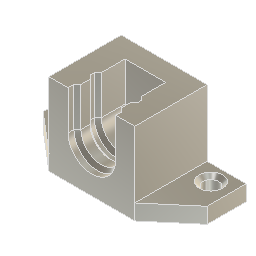
Крепление пневматического инструмента (Autodesk Fusion 360 design; units mm, degrees)
Autodesk Fusion 360 part; units mm, degrees
sketch "Sketch1" plane through (0, 0, 0) normal (0, 0, 1) x (1, 0, 0)
  line L0 (-5.9, 3.5) -> (-11, 3.5)
  line L1 (-11, 3.5) -> (-11, 22)
  line L2 (-11, 22) -> (0, 22)
  line L3 (5.9, 3.5) -> (11, 3.5)
  line L4 (11, 22) -> (0, 22)
  line L5 (11, 3.5) -> (11, 22)
  line L6 (-5.9, 3.5) -> (5.9, 3.5)
  line L7 (-6.1, 4.9828) -> (-6.1, 3.5)
  line L8 (-5.2, 5.8828) -> (-6.1, 4.9828)
  line L9 (-5.2, 8.2172) -> (-5.2, 5.8828)
  line L10 (-6.1, 9.1172) -> (-5.2, 8.2172)
  line L11 (-6.1, 9.1172) -> (-6.1, 10.1828)
  line L12 (-5.2, 11.0828) -> (-6.1, 10.1828)
  line L13 (-5.2, 16) -> (-5.2, 11.0828)
  line L14 (-5.2, 16) -> (-5.2, 17.2)
  line L15 (-5.2, 17.2) -> (0, 17.2)
  line L16 (5.2, 17.2) -> (0, 17.2)
  line L17 (5.2, 16) -> (5.2, 17.2)
  line L18 (5.2, 16) -> (5.2, 11.0828)
  line L19 (5.2, 11.0828) -> (6.1, 10.1828)
  line L20 (6.1, 9.1172) -> (6.1, 10.1828)
  line L21 (6.1, 9.1172) -> (5.2, 8.2172)
  line L22 (5.2, 8.2172) -> (5.2, 5.8828)
  line L23 (5.2, 5.8828) -> (6.1, 4.9828)
  line L24 (6.1, 4.9828) -> (6.1, 3.5)
  constraint perpendicular L0 L1
extrude "Extrude1" add sketch "Sketch1" along normal blind 5 contours L0 L1 L2 L3 L4 L5 L7 L8 L9 L10 L11 L12 L13 L14 L15 L16 L17 L18 L19 L20 L21 L22 L23 L24 makes body 1
extrude "Extrude2" add sketch "Sketch1" along normal blind 20 contours L0 L1 L2 L3 L4 L5 L7 L8 L9 L10 L11 L12 L13 L14 L15 L16 L17 L18 L19 L20 L21 L22 L23 L24 bodies 1
sketch "Sketch3" plane through (0, 0, 0) normal (0, 0, 1) x (1, 0, 0)
  line L0 (-5.2, 17.2) -> (-11, 17.2)
  line L1 (-6.1, 3.5) -> (-11, 3.5)
  line L2 (-11, 3.5) -> (-11, 17.2)
  line L3 (-6.1, 9.1172) -> (-6.1, 10.1828)
  line L4 (-5.2, 11.0828) -> (-6.1, 10.1828)
  line L5 (-5.2, 17.2) -> (-5.2, 11.0828)
  line L6 (-6.1, 4.9828) -> (-6.1, 3.5)
  line L7 (-5.2, 5.8828) -> (-6.1, 4.9828)
  line L8 (-5.2, 8.2172) -> (-5.2, 5.8828)
  line L9 (-6.1, 9.1172) -> (-5.2, 8.2172)
  constraint perpendicular L0 L2
revolve "Revolve1" add sketch "Sketch3" angle 360 about axis through (0, 1.75, 0) along (0, 1, 0) separate body makes body 2
sketch "Sketch4" plane through (0, 3.5, 0) normal (0, -1, 0) x (1, 0, 0)
  circle A0 centre (0, 0) radius 11
  circle A1 centre (0, 0) radius 6.1
sketch "Sketch5" plane through (0, 3.5, 0) normal (0, -1, 0) x (1, 0, 0)
  line L0 (-11, 0) -> (11, 0)
  line L1 (11, 0) -> (11, 12)
  line L2 (11, 12) -> (-11, 12)
  line L3 (-11, 12) -> (-11, 0)
  constraint horizontal L0
  constraint vertical L1
  constraint horizontal L2
  constraint vertical L3
extrude "Extrude3" cut sketch "Sketch5" against normal blind 25 bodies 2
sketch "Sketch6" plane through (0, 0, 0) normal (0, 0, -1) x (1, 0, 0)
  line L0 (-11, -3.5) -> (-11, -22)
  line L1 (-11, -22) -> (11, -22)
  line L2 (11, -22) -> (11, -3.5)
  line L3 (-6.1, -3.5) -> (-11, -3.5)
  line L4 (-11, -22) -> (11, -22)
  line L5 (11, -22) -> (11, -17.2)
  line L6 (11, -17.2) -> (-11, -17.2)
  line L7 (-11, -17.2) -> (-11, -22)
  line L8 (5.2, -8.2172) -> (6.1, -9.1172)
  line L9 (6.1, -9.1172) -> (6.1, -10.1828)
  line L10 (6.1, -10.1828) -> (5.2, -11.0828)
  line L11 (5.2, -11.0828) -> (5.2, -17.2)
  line L12 (5.2, -17.2) -> (-5.2, -17.2)
  line L13 (-5.2, -17.2) -> (-5.2, -11.0828)
  line L14 (-5.2, -11.0828) -> (-6.1, -10.1828)
  line L15 (-6.1, -10.1828) -> (-6.1, -9.1172)
  line L16 (-6.1, -9.1172) -> (-5.2, -8.2172)
  line L17 (-5.2, -8.2172) -> (-5.2, -5.8828)
  line L18 (-5.2, -5.8828) -> (-6.1, -4.9828)
  line L19 (-6.1, -4.9828) -> (-6.1, -3.5)
  line L20 (11, -3.5) -> (6.1, -3.5)
  line L21 (6.1, -3.5) -> (6.1, -4.9828)
  line L22 (6.1, -4.9828) -> (5.2, -5.8828)
  line L23 (5.2, -5.8828) -> (5.2, -8.2172)
  dimension "d40" = 4.8
  constraint horizontal L4
  constraint vertical L5
  constraint horizontal L6
  constraint vertical L7
  constraint coincident L2 L5.end
  constraint coincident L0.end L1.start
  measures "d40" distance of L1.end L5.end
extrude "Extrude4" add sketch "Sketch6" along normal blind 11 contours L0 L1 L2 L4 L5 L6 L7 L12 bodies 1
sketch "Sketch7" plane through (0, 0, 20) normal (0, 0, 1) x (-1, 0, 0)
  line L0 (-6.1, -3.5) -> (-11, -3.5)
  line L1 (-11, -3.5) -> (-11, -22)
  line L2 (-11, -22) -> (11, -22)
  line L3 (11, -22) -> (11, -3.5)
  line L4 (11, -22) -> (21, -22)
  line L5 (21, -22) -> (21, -12)
  line L6 (11, -12) -> (11, -22)
  line L7 (-11, -22) -> (-21, -22)
  line L8 (-21, -22) -> (-21, -12)
  line L9 (-11, -12) -> (-11, -22)
  circle A0 centre (16, -18) radius 2
  circle A1 centre (-16, -18) radius 2
  line L10 (-11, -3.5) -> (-11, -12)
  line L11 (21, -12) -> (11, -3.5)
  line L12 (-11, -3.5) -> (-21, -12)
  line L13 (-6.1, -9.1172) -> (-5.2, -8.2172)
  line L14 (-5.2, -5.8828) -> (-6.1, -4.9828)
  line L15 (-6.1, -4.9828) -> (-6.1, -3.5)
  line L16 (6.1, -3.5) -> (6.1, -4.9828)
  line L17 (6.1, -4.9828) -> (5.2, -5.8828)
  line L18 (5.2, -8.2172) -> (6.1, -9.1172)
  line L19 (6.1, -9.1172) -> (6.1, -10.1828)
  line L20 (6.1, -10.1828) -> (5.2, -11.0828)
  line L21 (-5.2, -11.0828) -> (-6.1, -10.1828)
  line L22 (-6.1, -10.1828) -> (-6.1, -9.1172)
  line L23 (11, -3.5) -> (6.1, -3.5)
  line L24 (-5.2, -8.2172) -> (-5.2, -5.8828)
  line L25 (5.2, -5.8828) -> (5.2, -8.2172)
  line L26 (5.2, -11.0828) -> (5.2, -17.2)
  line L27 (5.2, -17.2) -> (-5.2, -17.2)
  line L28 (-5.2, -17.2) -> (-5.2, -11.0828)
  dimension "d23" = 10
  dimension "d24" = 10
  dimension "d25" = 10
  dimension "d26" = 10
  dimension "d27" = 4
  dimension "d28" = 4
  dimension "d29" = 10
  constraint horizontal L4
  constraint vertical L5
  constraint vertical L6
  constraint coincident L2.end L3.start
  constraint horizontal L7
  constraint vertical L8
  constraint vertical L9
  constraint coincident L1.end L2.start
  constraint coincident L0.end L1.start
  constraint coincident L3.end L11.end
  measures "d23" distance of L2.end L4.end
  measures "d24" distance of L2.end L6.start
  measures "d25" distance of L1.end L7.end
  measures "d26" distance of L1.end L9.start
  measures "d27" diameter of A0
  measures "d28" diameter of A1
  measures "d29" distance of L4.end L5.end
extrude "Extrude6" add sketch "Sketch7" along normal blind -27 and the other way blind 31 contours L1 L7 L8 L9 L10 L12 | L3 L4 L5 L6 L11 bodies 1 2
chamfer "Chamfer2" distance 1 angle 45 2 edges at (-14.1353, 18.7232, -7) (17.8647, 18.7232, -7) on bodies 1
extrude "Extrude7" cut 1 faces at (-9.3667, 11.8943, 20) along direction (0, 0, -1) blind 10 on bodies 1 bodies 1 2
move_body "Move1" bodies 1 2 to x (1, 0, 0) y (0, 1, 0) z (0, 0, 1) at (0, 0, 11)
move_body "Move2" bodies 1 2 to x (1, 0, 0) y (0, 1, 0) z (0, 0, 1) at (0, -12, 0)
sketch "Sketch8" plane through (0, 5.2, 0) normal (0, -1, 0) x (1, 0, 0)
  line L0 (5.2, 21) -> (-5.2, 21)
  line L1 (-5.2, 21) -> (-5.2, 11)
  line L2 (-5.2, 11) -> (-11, 11)
  line L3 (-11, 11) -> (-11, 4)
  line L4 (-11, 4) -> (-11, 0)
  line L5 (-11, 0) -> (11, 0)
  line L6 (11, 0) -> (11, 4)
  line L7 (11, 4) -> (11, 11)
  line L8 (11, 11) -> (5.2, 11)
  line L9 (5.2, 11) -> (5.2, 21)
  arc A0 (-11, 11) -> (0, 0) centre (0, 11) ccw
  arc A1 (0, 0) -> (11, 11) centre (0, 11) ccw
  dimension "d41" = 11
  dimension "d42" = 11
  constraint coincident A0.end A1.start
  measures "d41" radius of A0
  measures "d42" radius of A1
extrude "Extrude8" add sketch "Sketch8" against normal blind 15 from surface at 13.7 contours L5 L6 L7 A1 | L3 L4 L5 A0 bodies 1 2
